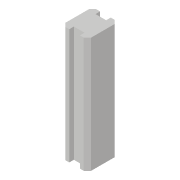
# Autodesk Inventor part: double slider
Saved by Autodesk Inventor 2018 (Build 220112000, 112)
## iProperties
Created: 2019-01-19
Part Number: double slider
Material: Generic
Document SubType Name: Modeling
Designer: ball
Density: 1 g/cm^3
Appearance: Default
Author: ball
Autodesk Inventor part; units mm, degrees
ref_plane "YZ Plane" through (0, 0, 0) normal (1, 0, 0) x (0, 1, 0)
ref_plane "XZ Plane" through (0, 0, 0) normal (0, 1, 0) x (-1, 0, 0)
ref_plane "XY Plane" through (0, 0, 0) normal (0, 0, 1) x (1, 0, 0)
sketch "Sketch1" plane through (0, 0, 0) normal (0, 1, 0) x (-1, 0, 0)
  line L0 (0, 0) -> (0, 3.1115)
  line L1 (0, 3.1115) -> (1.524, 3.1115)
  line L2 (1.524, 3.1115) -> (1.524, 4.4323)
  line L3 (1.524, 4.4323) -> (2.6416, 4.4323)
  line L4 (2.6416, 4.4323) -> (3.683, 3.4265)
  line L5 (3.683, 3.4265) -> (3.683, 0.0102)
  line L6 (7.9375, 0.0102) -> (-3.8699, 0.0102) construction
  line L7 (0, 0.0204) -> (0, -3.0911)
  line L8 (0, -3.0911) -> (1.524, -3.0911)
  line L9 (1.524, -3.0911) -> (1.524, -4.4119)
  line L10 (1.524, -4.4119) -> (2.6416, -4.4119)
  line L11 (2.6416, -4.4119) -> (3.683, -3.4061)
  line L12 (3.683, -3.4061) -> (3.683, 0.0102)
  line L13 (3.683, 3.4265) -> (3.683, -3.4061)
  line L14 (0, -3.0911) -> (0, 3.1115)
  line L15 (0, 3.1115) -> (-1.524, 3.1115)
  line L16 (-1.524, 3.1115) -> (-1.524, 4.4323)
  line L17 (-1.524, 4.4323) -> (-2.6416, 4.4323)
  line L18 (-2.6416, 4.4323) -> (-3.683, 3.4265)
  line L19 (-2.6416, -4.4119) -> (-3.683, -3.4061)
  line L20 (-1.524, -4.4119) -> (-2.6416, -4.4119)
  line L21 (-1.524, -3.0911) -> (-1.524, -4.4119)
  line L22 (0, -3.0911) -> (-1.524, -3.0911)
  line L23 (-3.683, 3.4265) -> (-3.683, -3.4061)
  dimension "d1" = 3.1115
  dimension "d2" = 1.524
  dimension "d3" = 1.3208
  dimension "d4" = 1.1176
  dimension "d5" = 1.4478
  dimension "d6" = 3.4163
  dimension "d7" = 3.683
  constraints: 48 end point, 14 symmetric about line, 3 perpendicular, 2 parallel, 1 collinear, 1 horizontal, 1 vertical
  measures "d1" distance of L0.start L0.end
  measures "d2" distance of L0.end L1.end
  measures "d3" distance of L1.end L2.end
  measures "d4" distance of L2.end L3.end
  measures "d5" distance of L3.end L4.end
  measures "d6" distance of L4.end L5.end
  measures "d7" distance between parallel lines of L0 L5
extrude "Extrusion1" add sketch "Sketch1" along normal blind 33.02
body "Solid1"
